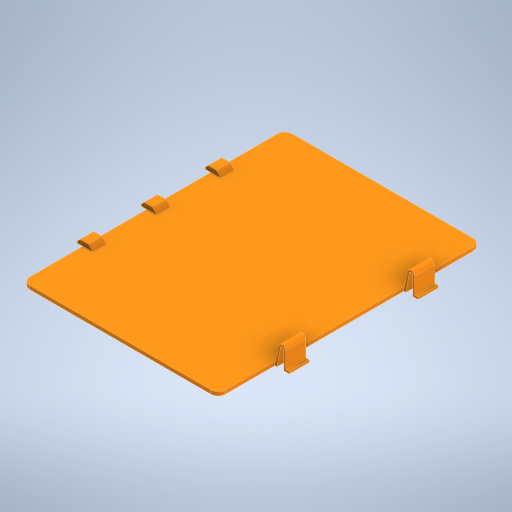
# Autodesk Inventor part: Toolbox cover
Saved by Autodesk Inventor 2023 (Build 270158000, 158)
## iProperties
Created: 2023-03-08
Part Number: Toolbox cover
Material: Типовые
Document SubType Name: Modeling
Designer: Josh
Density: 1 g/cm^3
Appearance: Оранжевый
Author: Josh
Autodesk Inventor part; units mm, degrees
ref_plane "YZ Plane" through (0, 0, 0) normal (1, 0, 0) x (0, 1, 0)
ref_plane "XZ Plane" through (0, 0, 0) normal (0, 1, 0) x (-1, 0, 0)
sketch "Эскиз1" plane through (0, 0, 0) normal (0, 1, 0) x (-1, 0, 0)
  line L0 (-49.5, -71.75) -> (49.5, -71.75)
  line L1 (53.5, -67.75) -> (53.5, 67.75)
  line L2 (49.5, 71.75) -> (-49.5, 71.75)
  line L3 (-53.5, 67.75) -> (-53.5, -67.75)
  line L4 (-53.5, -71.75) -> (53.5, 71.75) construction
  line L5 (53.5, -71.75) -> (-53.5, 71.75) construction
  arc A0 (53.5, 67.75) -> (49.5, 71.75) centre (49.5, 67.75) ccw
  arc A1 (49.5, -71.75) -> (53.5, -67.75) centre (49.5, -67.75) ccw
  arc A2 (-53.5, -67.75) -> (-49.5, -71.75) centre (-49.5, -67.75) ccw
  arc A3 (-49.5, 71.75) -> (-53.5, 67.75) centre (-49.5, 67.75) ccw
  line L6 (-53.5, 40.75) -> (-55.5, 40.75)
  line L7 (-55.5, 40.75) -> (-55.5, 29.75)
  line L8 (-55.5, 29.75) -> (-53.5, 29.75)
  line L9 (-53.5, 29.75) -> (-53.5, 40.75)
  line L10 (-53.5, 0) -> (53.5, 0)
  line L11 (-53.5, -40.75) -> (-55.5, -40.75)
  line L12 (-55.5, -40.75) -> (-55.5, -29.75)
  line L13 (-55.5, -29.75) -> (-53.5, -29.75)
  line L14 (-53.5, -29.75) -> (-53.5, -40.75)
  circle A4 centre (-30, -63.75) radius 2.05
  line L15 (0, -71.75) -> (0, 71.75)
  circle A5 centre (30, -63.75) radius 2.05
  circle A6 centre (-30, 63.75) radius 2.05
  circle A7 centre (30, 63.75) radius 2.05
  point P0 (0, 0)
  dimension "d0" = 107
  dimension "d1" = 143.5
  dimension "d2" = 4
  dimension "d3" = 2
  dimension "d4" = 11
  dimension "d5" = 31
  dimension "d6" = 4.1
  dimension "d7" = 8
  dimension "d8" = 60
  constraints: 32 end point, 9 point on line, 8 centre point, 8 point on circle, 8 tangent, 7 symmetric about line, 6 midpoint, 4 parallel, 3 equal radius, 2 horizontal, 2 perpendicular, 3 other
  measures "d0" distance of L5.end L4.end
  measures "d1" distance of L4.end L5.start
  measures "d2" radius of A0
  measures "d3" distance of L8.end L7.end
  measures "d4" distance of L7.end L6.end
  measures "d5" distance between parallel lines of L2 L6
  measures "d6" diameter of A4
  measures "d7" distance from line of L0 A4.centre
  measures "d8" distance of A5.centre A4.centre
extrude "Выдавливание1" add sketch "Эскиз1" along normal blind 2 contours A2 L3 L10 L15 L0 | L15 L10 L1 A1 L0 | L15 L2 A0 L1 L10 | L10 L3 A3 L2 L15 | A4 | A5 | A6 | A7
ref_plane "РабПлоскость1" through (-49.5, 0, 40.75) normal (0, 0, 1) x (1, 0, 0)
sketch "Эскиз3" plane through (-49.5, 0, 40.75) normal (0, 0, 1) x (1, 0, 0)
  line L0 (103, 0) -> (105.0373, 10.3941)
  arc A0 (109, 10.0094) -> (105.0373, 10.3941) centre (107, 10.0094) ccw
  line L1 (103, 2) -> (99, 2) projected
  line L2 (109, 10.0094) -> (109, 1.1)
  line L3 (104.1209, 0) -> (106.1168, 10.1825)
  arc A1 (107.9, 10.0094) -> (106.1168, 10.1825) centre (107, 10.0094) ccw
  line L4 (107.9, 10.0094) -> (107.9, 0)
  line L5 (103, 0) -> (99, 0) projected
  line L6 (103, 0) -> (104.1209, 0)
  line L7 (107.9, 0) -> (109, 0)
  line L8 (107.9, 0) -> (110.9, 0)
  line L9 (110.9, 0) -> (110.9, 1.1)
  line L10 (110.9, 1.1) -> (109, 1.1)
  line L11 (107.9, 1.1) -> (107.9, 0)
  line L12 (103, 2) -> (103.392, 2)
  line L13 (103, 2) -> (103, 0)
  point P0 (49.5, 0)
  point P1 (107.1933, 12)
  dimension "d19" = 10
  dimension "d20" = 2
  dimension "d21" = 6
  dimension "d22" = 1.1
  dimension "d23" = 1.1
  dimension "d24" = 1.1
  dimension "d25" = 3
  constraints: 24 end point, 5 point on circle, 3 horizontal, 3 tangent, 2 centre point, 2 parallel, 2 perpendicular, 1 collinear, 1 horizontal alignment, 1 point on line, 1 vertical
  measures "d19" vertical distance of point (107.193, 12) L1.start
  measures "d20" radius of A0
  measures "d21" distance from line of L1.start L2
  measures "d22" distance between parallel lines of L0 L3
  measures "d23" radial gap between concentric circles of A0 A1
  measures "d24" distance between parallel lines of L7 L10
  measures "d25" distance between parallel lines of L4 L9
extrude "Выдавливание2" add sketch "Эскиз3" against normal blind 11
mirror "Зеркальное отражение1" about plane through (0, 0, 0) normal (0, 0, 1) of "Выдавливание2"
sketch "Эскиз4" plane through (0, 2, 0) normal (0, 1, 0) x (1, 0, 0)
  line L0 (-48, -31.25) -> (-56.5, -31.25)
  line L1 (-56.5, -31.25) -> (-56.5, -38.75)
  line L2 (-56.5, -38.75) -> (-48, -38.75)
  line L3 (-48, -38.75) -> (-48, -31.25)
  line L4 (-53.5, 67.75) -> (-53.5, -67.75) projected
  line L5 (-49.5, -71.75) -> (49.5, -71.75) projected
  point P0 (0, 0)
  dimension "d28" = 7.5
  dimension "d29" = 3
  dimension "d30" = 33
  dimension "d31" = 5.5
  constraints: 8 end point, 2 parallel, 1 horizontal, 1 perpendicular
  measures "d28" distance between parallel lines of L2 L0
  measures "d29" distance between parallel lines of L1 L4
  measures "d30" distance between parallel lines of L5 L2
  measures "d31" distance between parallel lines of L3 L4
extrude "Выдавливание3" add sketch "Эскиз4" along normal blind 2.5
mirror "Зеркальное отражение2" about plane through (0, 0, 0) normal (0, 0, 1) of "Выдавливание3"
ref_plane "РабПлоскость3" through (-56.5, 2, 17.5) normal (0, 0, 1) x (1, 0, 0)
ref_plane "РабПлоскость2" through (-56.5, 2, 35) normal (0, 0, 1) x (1, 0, 0)
mirror "Зеркальное отражение3" about plane through (-56.5, 2, 17.5) normal (0, 0, 1) of "Выдавливание3"
chamfer "Фаска1" distance 1.5 angle 45 3 edges at (-56.5, 4.5, 35) (-56.5, 4.5, 0) (-56.5, 4.5, -35)
chamfer "Фаска2" distance 2.5 angle 45 3 edges at (-48, 4.5, 35) (-48, 4.5, -35) (-48, 4.5, 0)
